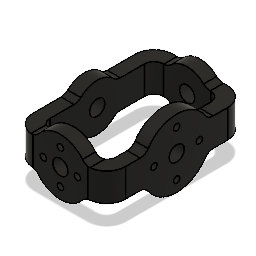
grt_cardan_joint_20190218 (Autodesk Fusion 360 design; units mm, degrees)
Autodesk Fusion 360 part; units mm, degrees
note: some values were not read from the file. Set by a fixed rule: which sketch regions a step uses.
sketch "Sketch" plane through (0, 0, 0) normal (0, 1, 0) x (-1, 0, 0)
  line L0 (-15.3985, -27.1047) -> (19.6015, -27.1047)
  line L1 (19.6015, -27.1047) -> (19.6015, 32.8953)
  line L2 (19.6015, 32.8953) -> (-15.3985, 32.8953)
  line L3 (-15.3985, 32.8953) -> (-15.3985, -27.1047)
  line L4 (-22.3985, 39.8953) -> (26.6015, 39.8953)
  line L5 (-22.3985, -34.1047) -> (-22.3985, 39.8953)
  line L6 (26.6015, 39.8953) -> (26.6015, -34.1047)
  line L7 (26.6015, -34.1047) -> (-22.3985, -34.1047)
  dimension "d1" = 60
  dimension "d2" = 35
  dimension "d3" = 7
  dimension "d4" = 7
  dimension "d5" = 7
  dimension "d6" = 7
  measures "d2" distance of L1
  measures "d3" distance of L1 L6
  measures "d4" distance of L2 L4
  measures "d5" distance of L3 L5
  measures "d6" distance of L0 L7
extrude "Extrude1" add sketch "Sketch" along normal blind 15
sketch "Sketch 1" plane through (0, 0, 0) normal (1, 0, 0) x (0, 0, -1)
sketch "Sketch 2" plane through (22.3985, 20.3985, 20.3985) normal (1, 0, 0) x (0, 0, -1)
  line L0 (-19.4968, -20.3985) -> (54.5032, -20.3985)
  line L1 (54.5032, -20.3985) -> (54.5032, -5.3985)
  line L2 (54.5032, -5.3985) -> (-19.4968, -5.3985)
  line L3 (-19.4968, -5.3985) -> (-19.4968, -20.3985)
  line L4 (-19.4968, -5.3985) -> (54.5032, -20.3985)
  line L5 (-19.4968, -20.3985) -> (54.5032, -5.3985)
  circle A0 centre (17.5032, -12.8985) radius 4
  circle A1 centre (17.5032, -12.8985) radius 18
  dimension "d9" = 8
  dimension "d30" = 36
  measures "d9" diameter of A0
  measures "d30" diameter of A1
extrude "Extrude2" cut sketch "Sketch 2" against normal up to surface (49 mm away) contours L4 L5 A0 | L4 L5 A0 | L4 L5 A0 | L4 L5 A0
sketch "Sketch 3" plane through (0, 0, 39.8953) normal (0, 0, 1) x (1, 0, 0)
  line L0 (-26.6015, 0) -> (22.3985, 0)
  line L1 (22.3985, 0) -> (22.3985, 15)
  line L2 (22.3985, 15) -> (-26.6015, 15)
  line L3 (-26.6015, 15) -> (-26.6015, 0)
  line L4 (-26.6015, 15) -> (22.3985, 0)
  line L5 (-26.6015, 0) -> (22.3985, 15)
  circle A0 centre (-2.1015, 7.5) radius 4
  circle A1 centre (-2.1015, 7.5) radius 15
  dimension "d12" = 8
  dimension "d22" = 30
  measures "d12" diameter of A0
  measures "d22" diameter of A1
extrude "Extrude3" cut sketch "Sketch 3" against normal up to surface (74 mm away) contours L4 L5 A0 | L4 L5 A0 | L4 L5 A0 | L4 L5 A0
extrude "Extrude4" add sketch "Sketch 2" against normal blind 7 contours L0 A1 | L2 A1
sketch "Sketch7" plane through (22.3985, 0, 0) normal (1, 0, 0) x (0, 0, -1)
  circle A0 centre (-2.8953, 7.5) radius 4
  line L0 (13.4678, 0) -> (34.1047, 0)
  line L1 (34.1047, 0) -> (34.1047, 15)
  line L2 (34.1047, 15) -> (13.4678, 15)
  arc A1 (13.4678, 15) -> (-19.2584, 15) centre (-2.8953, 7.5) ccw
  line L3 (-19.2584, 15) -> (-39.8953, 15)
  line L4 (-39.8953, 15) -> (-39.8953, 0)
  line L5 (-39.8953, 0) -> (-19.2584, 0)
  arc A2 (-19.2584, 0) -> (13.4678, 0) centre (-2.8953, 7.5) ccw
  line L6 (34.1047, 15) -> (-39.8953, 15)
  line L7 (-2.8953, 7.5) -> (-2.8953, 19.5)
  circle A3 centre (-2.8953, 19.5) radius 1.65
  circle A4 centre (-14.8953, 7.5) radius 1.65
  circle A5 centre (-2.8953, -4.5) radius 1.65
  circle A6 centre (9.1047, 7.5) radius 1.65
  dimension "d39" = 12
  dimension "d40" = 3.3
  dimension "d42" = 360
  measures "d40" diameter of A3
extrude "Extrude8" cut sketch "Sketch7" against normal up to surface (7 mm away) contours A3 | A4 | A5 | A6
sketch "Sketch 4" plane through (-26.6015, -24.6015, -24.6015) normal (-1, 0, 0) x (0, 0, 1)
  circle A0 centre (27.4968, 32.1015) radius 4
  line L0 (-9.5032, 24.6015) -> (64.4968, 24.6015)
  line L1 (64.4968, 24.6015) -> (64.4968, 39.6015)
  line L2 (64.4968, 39.6015) -> (-9.5032, 39.6015)
  line L3 (-9.5032, 39.6015) -> (-9.5032, 24.6015)
  circle A1 centre (27.4968, 32.1015) radius 12.5
  dimension "d19" = 25
  measures "d19" diameter of A1
extrude "Extrude5" add sketch "Sketch 4" against normal blind 7 contours L0 A1 | L2 A1
extrude "Extrude6" add sketch "Sketch 3" against normal blind 7 contours L0 A1 | L2 A1
sketch "Sketch 5" plane through (0, 0, -34.1047) normal (0, 0, -1) x (-1, 0, 0)
  circle A0 centre (2.1015, 7.5) radius 4
  line L0 (-22.3985, 0) -> (26.6015, 0)
  line L1 (26.6015, 0) -> (26.6015, 15)
  line L2 (26.6015, 15) -> (-22.3985, 15)
  line L3 (-22.3985, 15) -> (-22.3985, 0)
  circle A1 centre (2.1015, 7.5) radius 12.5
  dimension "d25" = 25
  measures "d25" diameter of A1
extrude "Extrude7" add sketch "Sketch 5" against normal blind 7 contours L0 A1 | L2 A1
fillet "Fillet1" radius 5 4 edges at (15.3985, 7.5, 32.8953) (-19.6015, 7.5, 32.8953) (-19.6015, 7.5, -27.1047) (15.3985, 7.5, -27.1047)
fillet "Fillet2" radius 10 4 edges at (-26.6015, 7.5, -34.1047) (22.3985, 7.5, -34.1047) (22.3985, 7.5, 39.8953) (-26.6015, 7.5, 39.8953)
fillet "Fillet3" radius 5 16 edges at (10.8888, 15, 36.3953) (18.8985, 15, 19.2584) (-23.1015, 15, 12.8953) (-23.1015, 15, -7.1047) (7.8985, 15, -30.6047) (18.8985, 15, -13.4678) (-12.1015, 15, -30.6047) (-15.0919, 15, 36.3953) (-23.1015, 0, -7.1047) (-12.1015, 0, -30.6047) (7.8985, 0, -30.6047) (18.8985, 0, -13.4678) (10.8888, 0, 36.3953) (18.8985, 0, 19.2584) (-15.0919, 0, 36.3953) (-23.1015, 0, 12.8953)
sketch "Sketch8" plane through (0, 0, 39.8953) normal (0, 0, 1) x (1, 0, 0)
  line L0 (-16.6015, 15.1253) -> (-16.6015, -0.1253)
  arc A0 (-13.8109, -1.875) -> (-16.6015, -0.1253) centre (-17.714, -5) ccw
  arc A1 (-13.8109, -1.875) -> (9.6078, -1.875) centre (-2.1015, 7.5) ccw
  arc A2 (12.3985, -0.1253) -> (9.6078, -1.875) centre (13.5109, -5) ccw
  line L1 (12.3985, -0.1253) -> (12.3985, 15.1253)
  arc A3 (9.6078, 16.875) -> (12.3985, 15.1253) centre (13.5109, 20) ccw
  arc A4 (9.6078, 16.875) -> (-13.8109, 16.875) centre (-2.1015, 7.5) ccw
  arc A5 (-16.6015, 15.1253) -> (-13.8109, 16.875) centre (-17.714, 20) ccw
  circle A6 centre (-2.1015, 7.5) radius 4
  line L2 (-2.1015, 7.5) -> (-2.1015, 16.5)
  dimension "d46" = 9
hole "Hole1" at (-2.1015, 16.5, 39.8953) direction (0, 0, -1) diameter 3.3 depth 20 tip angle 118
pattern_circular "C-Pattern1" count 4 over 360 about axis through (-2.1015, 7.5, 42.3953) along (0, 0, -1) of "Hole1"
